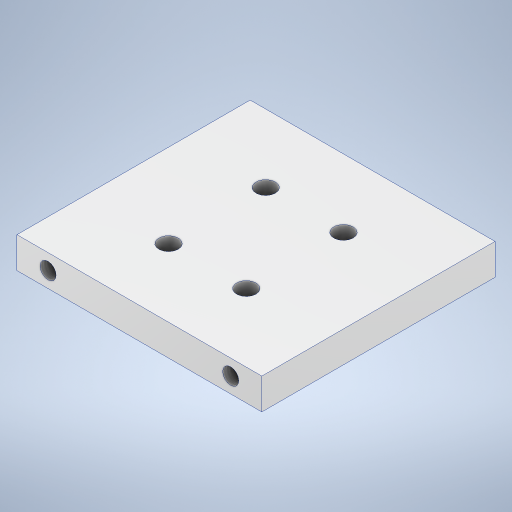
# Autodesk Inventor part: Traseira da caixa de sustentação
Saved by Autodesk Inventor 2023 (Build 270158000, 158)
## iProperties
Created: 2023-03-23
Part Number: Traseira da caixa de sustentação
Material: Aluminum 6061
Document SubType Name: Sheet Metal
Designer: 062190003
Density: 2.7 g/cm^3
Sheet Metal Rule: Default_mm
Appearance: Aluminum - Flat
Flat Pattern Width: 6.3 cm
Flat Pattern Length: 7.3 cm
Flat Pattern Area: 45.99 cm^2
Sheet Metal Width: 63,000 mm
Sheet Metal Length: 73,000 mm
Sheet Metal Area: 4599,000 mm^2
Author: 062190003
Autodesk Inventor part; units mm, degrees
ref_plane "YZ Plane" through (0, 0, 0) normal (1, 0, 0) x (0, 1, 0)
ref_plane "XZ Plane" through (0, 0, 0) normal (0, 1, 0) x (-1, 0, 0)
ref_plane "XY Plane" through (0, 0, 0) normal (0, 0, 1) x (1, 0, 0)
sketch "Sketch5" plane through (0, 0, 0) normal (0, 1, 0) x (-1, 0, 0)
  line L0 (0, 0) -> (63, 0)
  line L1 (63, 0) -> (63, -60)
  line L2 (63, -60) -> (0, -60)
  line L3 (0, -60) -> (0, 0)
  dimension "d68" = 63
  dimension "d69" = 60
  constraints: 8 end point, 2 parallel, 1 horizontal, 1 perpendicular
  measures "d68" distance of L1.end L2.end
  measures "d69" distance of L0.end L1.end
extrude "Extrusion2" add sketch "Sketch5" along normal blind 8
sketch "Sketch6" plane through (0, 8, 0) normal (0, 1, 0) x (1, 0, 0)
  line L0 (-63, 60) -> (-63, 0) projected
  line L1 (0, 60) -> (-63, 60) projected
  point P0 (0, 0)
  point P1 (-41.5, 42.5)
  point P2 (-41.5, 17.5)
  point P3 (-21.5, 42.5)
  point P4 (-21.5, 17.5)
  dimension "d74" = 25
  dimension "d77" = 20
  dimension "d80" = 63
  dimension "d81" = 60
  dimension "d82" = 21.5
  dimension "d83" = 17.5
  constraints: 1 horizontal, 1 vertical, 3 other
  measures "d74" distance of point (-41.5, 42.5) point (-41.5, 17.5)
  measures "d77" distance of point (-41.5, 42.5) point (-21.5, 42.5)
  measures "d80" distance of L1.start L0.start
  measures "d81" distance of L0.start L0.end
  measures "d82" distance from line of L0 point (-41.5, 42.5)
  measures "d83" distance from line of L1 point (-41.5, 42.5)
hole "Hole3" at (-41.5, 8, -42.5) at (-41.5, 8, -17.5) at (-21.5, 8, -42.5) at (-21.5, 8, -17.5) direction (0, -1, 0) diameter 5 end through all
sketch "Sketch7" plane through (-63, 0, 0) normal (0, 0, 1) x (1, 0, 0)
  line L0 (0, 0) -> (0, 8) projected
  line L1 (63, 0) -> (63, 8) projected
  point P0 (55, 4)
  point P1 (8, 4)
  point P2 (0, 4)
  dimension "d91" = 8
  dimension "d92" = 8
  constraints: 1 midpoint
  measures "d91" distance of point (0, 4) point (8, 4)
  measures "d92" distance from line of L1 point (55, 4)
hole "Hole4" at (-8, 4, 0) at (-55, 4, 0) direction (0, 0, -1) diameter 4.134 depth 14.2 tip angle 118 thread size "M5x0.8" class "6H" standard "ISO Metric profile"
sketch "Sketch8" plane through (0, 0, -60) normal (0, 0, -1) x (-1, 0, 0)
  circle A0 centre (8, 4) radius 2.067 projected
  circle A1 centre (55, 4) radius 2.067 projected
  point P0 (0, 0)
  constraints: 2 coincident
hole "Hole5" at (-8, 4, -60) at (-55, 4, -60) direction (0, 0, 1) diameter 4.134 depth 14.2 tip angle 118 thread size "M5x0.8" class "6H" standard "ISO Metric profile"
equation "\"d82\" = -0.5 * d77 + 0.5 * d80"
equation "\"d83\" = -0.5 * d74 + 0.5 * d81"
equation "\"d89\" = Thickness"
equation "\"BendRadius\" = Thickness"
equation "\"BendReliefWidth\" = Thickness"
equation "\"BendReliefDepth\" = 0.5 * Thickness"
equation "\"TransitionRadius\" = BendRadius"
equation "\"JacobiRadiusSize\" = BendRadius"
equation "\"GapSize\" = Thickness"
equation "\"Thickness\" = 5"
body "Solid3"
